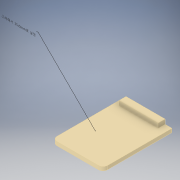
# Autodesk Inventor part: Case_Top
Saved by Autodesk Inventor 2020 (Build 240168000, 168)
## iProperties
Created: 2019-02-21
Part Number: Case_Top
Material: 일반
Document SubType Name: Modeling
Designer: Jeong Ji Hoon
Density: 1 g/cm^3
Appearance: 베이지색
Author: Jeong Ji Hoon
## iProperties of the stored document _3D 인쇄.ipt
Created: 2019-11-26
Part Number: _3D 인쇄
Material: 일반
Document SubType Name: Modeling
Designer: Knowblesse
Density: 1 g/cm^3
Appearance: 기본값
Author: Knowblesse
Autodesk Inventor part; units mm, degrees
ref_plane "YZ Plane" through (0, 0, 0) normal (1, 0, 0) x (0, 1, 0)
ref_plane "XZ Plane" through (0, 0, 0) normal (0, 1, 0) x (-1, 0, 0)
ref_plane "XY Plane" through (0, 0, 0) normal (0, 0, 1) x (1, 0, 0)
sketch "스케치1" plane through (0, 0, 0) normal (0, 1, 0) x (-1, 0, 0)
  line L0 (0, 0) -> (11, 0)
  line L1 (11, 0) -> (11, -15)
  line L2 (11, -15) -> (0, -15)
  line L3 (0, -15) -> (0, 0)
  dimension "d0" = 11
  dimension "d1" = 15
  constraints: 8 end point, 2 parallel, 1 horizontal, 1 perpendicular
  measures "d0" distance of L1.end L2.end
  measures "d1" distance of L0.end L1.end
extrude "돌출1" add sketch "스케치1" along normal blind 0.8
fillet "모깎기1" radius 1 2 edges at (0, 0.4, 0) (-11, 0.4, 0)
sketch "스케치2" plane through (0, 0.8, 0) normal (0, 1, 0) x (1, 0, 0)
  line L0 (0, 1) -> (0, 15) projected
  line L1 (0, 15) -> (-11, 15) projected
  line L2 (-1.5, 15) -> (-10, 15)
  line L3 (-10, 15) -> (-10, 13.5)
  line L4 (-10, 13.5) -> (-1.5, 13.5)
  line L5 (-1.5, 13.5) -> (-1.5, 15)
  point P0 (0, 0)
  dimension "d5" = 8.5
  dimension "d6" = 1.5
  dimension "d7" = 1.5
  constraints: 8 end point, 2 parallel, 1 collinear, 1 horizontal, 1 perpendicular
  measures "d5" distance of L4.end L3.end
  measures "d6" distance of L3.end L2.end
  measures "d7" distance between parallel lines of L0 L5
extrude "돌출2" add sketch "스케치2" along normal blind 1
